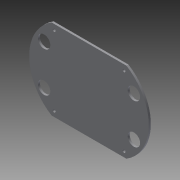
# Autodesk Inventor part: base
Saved by Autodesk Inventor 2015 (Build 190159000, 159)
## iProperties
Created: 2014-09-21
Part Number: base
Material: Générique
Document SubType Name: Modeling
Designer: astralien3000
Density: 1 g/cm^3
Appearance: Par défaut
Author: astralien3000
Autodesk Inventor part; units mm, degrees
ref_plane "YZ Plane" through (0, 0, 0) normal (1, 0, 0) x (0, 1, 0)
ref_plane "XZ Plane" through (0, 0, 0) normal (0, 1, 0) x (-1, 0, 0)
ref_plane "XY Plane" through (0, 0, 0) normal (0, 0, 1) x (1, 0, 0)
sketch "Esquisse1" plane through (0, 0, 0) normal (0, 1, 0) x (-1, 0, 0)
  circle A0 centre (0, 0) radius 25 construction
  line L0 (-25, 0) -> (25, 0) construction
  arc A1 (-75, -80.7775) -> (-75, 80.7775) centre (-25, 0) ccw construction
  arc A2 (75, 80.7775) -> (75, -80.7775) centre (25, 0) ccw construction
  line L1 (0, 25) -> (0, 0) construction
  line L2 (-75, 80.7775) -> (75, 80.7775)
  line L3 (-75, -80.7775) -> (75, -80.7775)
  arc A3 (75, -80.7775) -> (75, 80.7775) centre (25, 0) ccw
  arc A4 (-75, 80.7775) -> (-75, -80.7775) centre (-25, 0) ccw
  dimension "d0" = 50
  dimension "d1" = 190
  dimension "d2" = 150
  constraints: 11 point on circle, 8 end point, 5 centre point, 3 coincident, 2 perpendicular, 1 horizontal, 1 midpoint, 2 other
  measures "d0" diameter of A0
  measures "d1" diameter of A1
  measures "d2" distance of L2.start L2.end
extrude "Extrusion1" add sketch "Esquisse1" along normal blind 4
sketch "Esquisse16" plane through (0, 0, 0) normal (0, -1, 0) x (1, 0, 0)
  line L0 (-70, 70) -> (70, 70) construction
  line L1 (70, 70) -> (70, -70) construction
  line L2 (70, -70) -> (-70, -70) construction
  line L3 (-70, -70) -> (-70, 70) construction
  circle A0 centre (70, 70) radius 3
  circle A1 centre (-70, 70) radius 3
  circle A2 centre (-70, -70) radius 3
  circle A3 centre (70, -70) radius 3
  point P0 (0, 0)
  dimension "d146" = 140
  dimension "d147" = 140
  dimension "d148" = 6
  dimension "d149" = 6
  dimension "d150" = 6
  dimension "d151" = 6
  dimension "d152" = 70
  dimension "d153" = 70
  constraints: 8 end point, 4 centre point, 4 coincident, 2 parallel, 1 horizontal, 1 perpendicular
  measures "d146" distance between parallel lines of L3 L1
  measures "d147" distance of L0.end L1.end
  measures "d148" diameter of A1
  measures "d149" diameter of A0
  measures "d150" diameter of A3
  measures "d151" diameter of A2
  measures "d152" distance from line of point (0, 0) L1
  measures "d153" distance from line of point (0, 0) L0
extrude "Extrusion13" cut sketch "Esquisse16" against normal through all
sketch "Esquisse18" plane through (0, 0, 0) normal (0, -1, 0) x (1, 0, 0)
  line L0 (-90, 40) -> (90, 40) construction
  line L1 (90, 40) -> (90, -40) construction
  line L2 (90, -40) -> (-90, -40) construction
  line L3 (-90, -40) -> (-90, 40) construction
  circle A0 centre (-90, 40) radius 12.5
  circle A1 centre (90, 40) radius 12.5
  circle A2 centre (90, -40) radius 12.5
  circle A3 centre (-90, -40) radius 12.5
  point P0 (0, 0)
  dimension "d170" = 180
  dimension "d171" = 90
  dimension "d172" = 80
  dimension "d173" = 40
  dimension "d174" = 25
  dimension "d175" = 25
  dimension "d176" = 25
  dimension "d177" = 25
  constraints: 8 end point, 4 centre point, 4 coincident, 2 parallel, 1 horizontal, 1 perpendicular
  measures "d170" distance of L0.start L0.end
  measures "d171" distance from line of L1 point (0, 0)
  measures "d172" distance of L0.end L1.end
  measures "d173" distance from line of point (0, 0) L0
  measures "d174" diameter of A3
  measures "d175" diameter of A0
  measures "d176" diameter of A1
  measures "d177" diameter of A2
extrude "Extrusion15" cut sketch "Esquisse18" against normal through all
